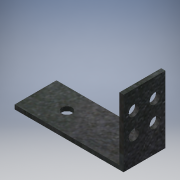
# Autodesk Inventor part: motorBracket
Saved by Autodesk Inventor 2016 (Build 200138000, 138)
## iProperties
Created: 2015-11-15
Part Number: motorBracket
Material: Steel
Document SubType Name: Modeling
Designer: Artur
Density: 7.85 g/cm^3
Appearance: Plate
Mass: 20.144 g
Surface Area: 81.9215 cm^2
Volume: 7.46073 cm^3
Author: Artur
Autodesk Inventor part; units mm, degrees
ref_plane "YZ Plane" through (0, 0, 0) normal (1, 0, 0) x (0, 1, 0)
ref_plane "XZ Plane" through (0, 0, 0) normal (0, 1, 0) x (-1, 0, 0)
ref_plane "XY Plane" through (0, 0, 0) normal (0, 0, 1) x (1, 0, 0)
sketch "Sketch1" plane through (0, 0, 0) normal (0, 1, 0) x (-1, 0, 0)
  line L0 (0, 0) -> (0, -32)
  line L1 (0, -32) -> (52, -32)
  line L2 (52, -32) -> (52, -30)
  line L3 (52, -30) -> (2, -30)
  line L4 (2, -30) -> (2, 0)
  line L5 (2, 0) -> (0, 0)
  dimension "d0" = 2
  dimension "d1" = 2
  dimension "d2" = 50
  dimension "d3" = 30
  constraints: 12 end point, 5 perpendicular, 1 vertical
  measures "d0" distance of L4.end L0.start
  measures "d1" distance of L1.end L2.end
  measures "d2" distance of L2.end L3.end
  measures "d3" distance of L3.end L4.end
extrude "base" add sketch "Sketch1" along normal blind 20
sketch "Sketch2" plane through (-52, 0, -30) normal (0, 0, 1) x (1, 0, 0)
  line L0 (0, 0) -> (50, 0) construction
  line L1 (50, 0) -> (50, 20) construction
  line L2 (0, 20) -> (50, 20) construction
  line L3 (0, 0) -> (0, 20) construction
  line L4 (0, 0) -> (50, 0) construction
  line L5 (52, 20) -> (0, 20) construction
  circle A0 centre (15, 10) radius 2.5
  line L6 (0, 0) -> (0, 20) projected
  line L7 (0, 10) -> (52, 10)
  line L8 (52, 0) -> (52, 20) projected
  dimension "d6" = 5
  dimension "d9" = 15
  constraints: 2 end point, 2 midpoint, 1 centre point, 1 point on line
  measures "d6" diameter of A0
  measures "d9" distance from line of L3 A0.centre
extrude "shaftHole" cut sketch "Sketch2" against normal blind 30
sketch "Sketch4" plane through (0, 0, 0) normal (1, 0, 0) x (0, 0, -1)
  line L0 (32, 0) -> (32, 20) construction
  line L1 (0, 0) -> (0, 20) construction
  line L2 (30, 0) -> (30, 20) construction
  line L3 (0, 10) -> (30, 10) construction
  line L4 (9, 5) -> (9, 15) construction
  line L5 (19, 15) -> (19, 5) construction
  point P0 (9, 10)
  point P1 (19, 10)
  dimension "d22" = 30
  dimension "d29" = 10
  dimension "d30" = 9
  dimension "d31" = 10
  dimension "d32" = 10
  constraints: 6 end point, 4 coincident, 4 midpoint, 2 point on line, 2 vertical
  measures "d22" distance of L3.start L3.end
  measures "d29" distance of L4.start L4.end
  measures "d30" distance between parallel lines of L1 L4
  measures "d31" distance of L5.start L5.end
  measures "d32" distance between parallel lines of L4 L5
hole "Hole1" at (0, 5, -9) at (0, 15, -9) at (0, 15, -19) at (0, 5, -19) direction (-1, 0, 0) diameter 5 end through all
equation "\"d1\" = d0"
equation "\"d31\" = d29"
body "Solid1"
